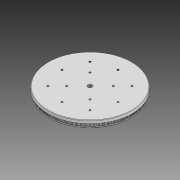
# Autodesk Inventor part: Turntable
Saved by Autodesk Inventor 2020 (Build 240168000, 168)
## iProperties
Created: 2020-10-19
Part Number: Turntable
Material: Generic
Document SubType Name: Modeling
Designer: DDeGo
Density: 1 g/cm^3
Appearance: Default
Author: DDeGo
Autodesk Inventor part; units mm, degrees
ref_plane "YZ Plane" through (0, 0, 0) normal (1, 0, 0) x (0, 1, 0)
ref_plane "XZ Plane" through (0, 0, 0) normal (0, 1, 0) x (-1, 0, 0)
ref_plane "XY Plane" through (0, 0, 0) normal (0, 0, 1) x (1, 0, 0)
sketch "Sketch1" plane through (0, 0, 0) normal (0, 0, 1) x (1, 0, 0)
  line L0 (0, 0) -> (0, 13.2) construction
  line L1 (0, 14.7) -> (90, 14.7)
  line L2 (88.5, 0) -> (73.1, 0)
  line L3 (73.1, 0) -> (73.1, 12.8)
  line L4 (0, 0) -> (73.1, 0) construction
  line L5 (0, 13.2) -> (0, 14.7)
  line L6 (90, 8.5) -> (87.5, 8.5)
  line L7 (87.5, 8.5) -> (87.5, 1.5)
  line L8 (87.5, 1.5) -> (88.5, 1.5)
  line L9 (90, 14.7) -> (90, 8.5)
  line L10 (88.5, 1.5) -> (88.5, 0)
  line L11 (73.1, 12.8) -> (69.1, 12.8)
  line L12 (69.1, 12.8) -> (69.1, 13.2)
  line L13 (69.1, 13.2) -> (0, 13.2)
  dimension "d0" = 90
  dimension "d6" = 7
  dimension "d9" = 87.5
  dimension "d11" = 1
  dimension "d12" = 1.5
  dimension "d13" = 73.1
  dimension "d14" = 12.8
  dimension "d15" = 0.4
  dimension "d16" = 4
  dimension "d17" = 1.5
  constraints: 28 end point, 9 perpendicular, 3 horizontal, 2 vertical, 1 collinear, 1 parallel
  measures "d0" distance of L1.start L1.end
  measures "d6" distance of L6.end L7.end
  measures "d9" distance between parallel lines of L7 L0
  measures "d11" distance of L7.end L8.end
  measures "d12" distance of L8.end L2.start
  measures "d13" distance between parallel lines of L0 L3
  measures "d14" distance of L2.end L3.end
  measures "d15" distance of L11.end L12.end
  measures "d16" distance of L3.end L11.end
  measures "d17" distance between parallel lines of L1 L13
revolve "Revolution1" add sketch "Sketch1" angle 360 about axis through (0, 13.2, 0) along (0, 1, 0)
sketch "Sketch3" plane through (0, 8.5, 0) normal (0, -1, 0) x (1, 0, 0)
  line L0 (0, 0) -> (87.5, 0) construction
  circle A0 centre (0, 0) radius 87.5 projected
  circle A1 centre (87.5, 0) radius 0.65
  circle A2 centre (87.478, -1.9633) radius 0.65
  circle A3 centre (87.4119, -3.9257) radius 0.65
  circle A4 centre (87.3018, -5.886) radius 0.65
  circle A5 centre (87.1478, -7.8434) radius 0.65
  circle A6 centre (86.9498, -9.7969) radius 0.65
  circle A7 centre (86.7081, -11.7454) radius 0.65
  circle A8 centre (86.4227, -13.688) radius 0.65
  circle A9 centre (86.0938, -15.6237) radius 0.65
  circle A10 centre (85.7216, -17.5516) radius 0.65
  circle A11 centre (85.3062, -19.4706) radius 0.65
  circle A12 centre (84.8478, -21.3798) radius 0.65
  circle A13 centre (84.3468, -23.2782) radius 0.65
  circle A14 centre (83.8032, -25.1649) radius 0.65
  circle A15 centre (83.2174, -27.039) radius 0.65
  circle A16 centre (82.5898, -28.8994) radius 0.65
  circle A17 centre (81.9206, -30.7453) radius 0.65
  circle A18 centre (81.2101, -32.5757) radius 0.65
  circle A19 centre (80.4587, -34.3897) radius 0.65
  circle A20 centre (79.6668, -36.1864) radius 0.65
  circle A21 centre (78.8348, -37.9648) radius 0.65
  circle A22 centre (77.9631, -39.7242) radius 0.65
  circle A23 centre (77.0521, -41.4635) radius 0.65
  circle A24 centre (76.1023, -43.182) radius 0.65
  circle A25 centre (75.1143, -44.8787) radius 0.65
  circle A26 centre (74.0884, -46.5528) radius 0.65
  circle A27 centre (73.0252, -48.2035) radius 0.65
  circle A28 centre (71.9252, -49.8299) radius 0.65
  circle A29 centre (70.789, -51.4312) radius 0.65
  circle A30 centre (69.6171, -53.0066) radius 0.65
  circle A31 centre (68.4103, -54.5554) radius 0.65
  circle A32 centre (67.1689, -56.0766) radius 0.65
  circle A33 centre (65.8938, -57.5696) radius 0.65
  circle A34 centre (64.5854, -59.0337) radius 0.65
  circle A35 centre (63.2446, -60.468) radius 0.65
  circle A36 centre (61.8718, -61.8718) radius 0.65
  circle A37 centre (60.468, -63.2446) radius 0.65
  circle A38 centre (59.0337, -64.5854) radius 0.65
  circle A39 centre (57.5696, -65.8938) radius 0.65
  circle A40 centre (56.0766, -67.1689) radius 0.65
  circle A41 centre (54.5554, -68.4103) radius 0.65
  circle A42 centre (53.0066, -69.6171) radius 0.65
  circle A43 centre (51.4312, -70.789) radius 0.65
  circle A44 centre (49.8299, -71.9252) radius 0.65
  circle A45 centre (48.2035, -73.0252) radius 0.65
  circle A46 centre (46.5528, -74.0884) radius 0.65
  circle A47 centre (44.8787, -75.1143) radius 0.65
  circle A48 centre (43.182, -76.1023) radius 0.65
  circle A49 centre (41.4635, -77.0521) radius 0.65
  circle A50 centre (39.7242, -77.9631) radius 0.65
  circle A51 centre (37.9648, -78.8348) radius 0.65
  circle A52 centre (36.1864, -79.6668) radius 0.65
  circle A53 centre (34.3897, -80.4587) radius 0.65
  circle A54 centre (32.5757, -81.2101) radius 0.65
  circle A55 centre (30.7453, -81.9206) radius 0.65
  circle A56 centre (28.8994, -82.5898) radius 0.65
  circle A57 centre (27.039, -83.2174) radius 0.65
  circle A58 centre (25.1649, -83.8032) radius 0.65
  circle A59 centre (23.2782, -84.3468) radius 0.65
  circle A60 centre (21.3798, -84.8478) radius 0.65
  circle A61 centre (19.4706, -85.3062) radius 0.65
  circle A62 centre (17.5516, -85.7216) radius 0.65
  circle A63 centre (15.6237, -86.0938) radius 0.65
  circle A64 centre (13.688, -86.4227) radius 0.65
  circle A65 centre (11.7454, -86.7081) radius 0.65
  circle A66 centre (9.7969, -86.9498) radius 0.65
  circle A67 centre (7.8434, -87.1478) radius 0.65
  circle A68 centre (5.886, -87.3018) radius 0.65
  circle A69 centre (3.9257, -87.4119) radius 0.65
  circle A70 centre (1.9633, -87.478) radius 0.65
  circle A71 centre (0, -87.5) radius 0.65
  circle A72 centre (-1.9633, -87.478) radius 0.65
  circle A73 centre (-3.9257, -87.4119) radius 0.65
  circle A74 centre (-5.886, -87.3018) radius 0.65
  circle A75 centre (-7.8434, -87.1478) radius 0.65
  circle A76 centre (-9.7969, -86.9498) radius 0.65
  circle A77 centre (-11.7454, -86.7081) radius 0.65
  circle A78 centre (-13.688, -86.4227) radius 0.65
  circle A79 centre (-15.6237, -86.0938) radius 0.65
  circle A80 centre (-17.5516, -85.7216) radius 0.65
  circle A81 centre (-19.4706, -85.3062) radius 0.65
  circle A82 centre (-21.3798, -84.8478) radius 0.65
  circle A83 centre (-23.2782, -84.3468) radius 0.65
  circle A84 centre (-25.1649, -83.8032) radius 0.65
  circle A85 centre (-27.039, -83.2174) radius 0.65
  circle A86 centre (-28.8994, -82.5898) radius 0.65
  circle A87 centre (-30.7453, -81.9206) radius 0.65
  circle A88 centre (-32.5757, -81.2101) radius 0.65
  circle A89 centre (-34.3897, -80.4587) radius 0.65
  circle A90 centre (-36.1864, -79.6668) radius 0.65
  circle A91 centre (-37.9648, -78.8348) radius 0.65
  circle A92 centre (-39.7242, -77.9631) radius 0.65
  circle A93 centre (-41.4635, -77.0521) radius 0.65
  circle A94 centre (-43.182, -76.1023) radius 0.65
  circle A95 centre (-44.8787, -75.1143) radius 0.65
  circle A96 centre (-46.5528, -74.0884) radius 0.65
  circle A97 centre (-48.2035, -73.0252) radius 0.65
  circle A98 centre (-49.8299, -71.9252) radius 0.65
  circle A99 centre (-51.4312, -70.789) radius 0.65
  circle A100 centre (-53.0066, -69.6171) radius 0.65
  circle A101 centre (-54.5554, -68.4103) radius 0.65
  circle A102 centre (-56.0766, -67.1689) radius 0.65
  circle A103 centre (-57.5696, -65.8938) radius 0.65
  circle A104 centre (-59.0337, -64.5854) radius 0.65
  circle A105 centre (-60.468, -63.2446) radius 0.65
  circle A106 centre (-61.8718, -61.8718) radius 0.65
  circle A107 centre (-63.2446, -60.468) radius 0.65
  circle A108 centre (-64.5854, -59.0337) radius 0.65
  circle A109 centre (-65.8938, -57.5696) radius 0.65
  circle A110 centre (-67.1689, -56.0766) radius 0.65
  circle A111 centre (-68.4103, -54.5554) radius 0.65
  circle A112 centre (-69.6171, -53.0066) radius 0.65
  circle A113 centre (-70.789, -51.4312) radius 0.65
  circle A114 centre (-71.9252, -49.8299) radius 0.65
  circle A115 centre (-73.0252, -48.2035) radius 0.65
  circle A116 centre (-74.0884, -46.5528) radius 0.65
  circle A117 centre (-75.1143, -44.8787) radius 0.65
  circle A118 centre (-76.1023, -43.182) radius 0.65
  circle A119 centre (-77.0521, -41.4635) radius 0.65
  circle A120 centre (-77.9631, -39.7242) radius 0.65
  circle A121 centre (-78.8348, -37.9648) radius 0.65
  circle A122 centre (-79.6668, -36.1864) radius 0.65
  circle A123 centre (-80.4587, -34.3897) radius 0.65
  circle A124 centre (-81.2101, -32.5757) radius 0.65
  circle A125 centre (-81.9206, -30.7453) radius 0.65
  circle A126 centre (-82.5898, -28.8994) radius 0.65
  circle A127 centre (-83.2174, -27.039) radius 0.65
  circle A128 centre (-83.8032, -25.1649) radius 0.65
  circle A129 centre (-84.3468, -23.2782) radius 0.65
  circle A130 centre (-84.8478, -21.3798) radius 0.65
  circle A131 centre (-85.3062, -19.4706) radius 0.65
  circle A132 centre (-85.7216, -17.5516) radius 0.65
  circle A133 centre (-86.0938, -15.6237) radius 0.65
  circle A134 centre (-86.4227, -13.688) radius 0.65
  circle A135 centre (-86.7081, -11.7454) radius 0.65
  circle A136 centre (-86.9498, -9.7969) radius 0.65
  circle A137 centre (-87.1478, -7.8434) radius 0.65
  circle A138 centre (-87.3018, -5.886) radius 0.65
  circle A139 centre (-87.4119, -3.9257) radius 0.65
  circle A140 centre (-87.478, -1.9633) radius 0.65
  circle A141 centre (-87.5, 0) radius 0.65
  circle A142 centre (-87.478, 1.9633) radius 0.65
  circle A143 centre (-87.4119, 3.9257) radius 0.65
  circle A144 centre (-87.3018, 5.886) radius 0.65
  circle A145 centre (-87.1478, 7.8434) radius 0.65
  circle A146 centre (-86.9498, 9.7969) radius 0.65
  circle A147 centre (-86.7081, 11.7454) radius 0.65
  circle A148 centre (-86.4227, 13.688) radius 0.65
  circle A149 centre (-86.0938, 15.6237) radius 0.65
  circle A150 centre (-85.7216, 17.5516) radius 0.65
  circle A151 centre (-85.3062, 19.4706) radius 0.65
  circle A152 centre (-84.8478, 21.3798) radius 0.65
  circle A153 centre (-84.3468, 23.2782) radius 0.65
  circle A154 centre (-83.8032, 25.1649) radius 0.65
  circle A155 centre (-83.2174, 27.039) radius 0.65
  circle A156 centre (-82.5898, 28.8994) radius 0.65
  circle A157 centre (-81.9206, 30.7453) radius 0.65
  circle A158 centre (-81.2101, 32.5757) radius 0.65
  circle A159 centre (-80.4587, 34.3897) radius 0.65
  circle A160 centre (-79.6668, 36.1864) radius 0.65
  circle A161 centre (-78.8348, 37.9648) radius 0.65
  circle A162 centre (-77.9631, 39.7242) radius 0.65
  circle A163 centre (-77.0521, 41.4635) radius 0.65
  circle A164 centre (-76.1023, 43.182) radius 0.65
  circle A165 centre (-75.1143, 44.8787) radius 0.65
  circle A166 centre (-74.0884, 46.5528) radius 0.65
  circle A167 centre (-73.0252, 48.2035) radius 0.65
  circle A168 centre (-71.9252, 49.8299) radius 0.65
  circle A169 centre (-70.789, 51.4312) radius 0.65
  circle A170 centre (-69.6171, 53.0066) radius 0.65
  circle A171 centre (-68.4103, 54.5554) radius 0.65
  circle A172 centre (-67.1689, 56.0766) radius 0.65
  circle A173 centre (-65.8938, 57.5696) radius 0.65
  circle A174 centre (-64.5854, 59.0337) radius 0.65
  circle A175 centre (-63.2446, 60.468) radius 0.65
  circle A176 centre (-61.8718, 61.8718) radius 0.65
  circle A177 centre (-60.468, 63.2446) radius 0.65
  circle A178 centre (-59.0337, 64.5854) radius 0.65
  circle A179 centre (-57.5696, 65.8938) radius 0.65
  circle A180 centre (-56.0766, 67.1689) radius 0.65
  circle A181 centre (-54.5554, 68.4103) radius 0.65
  circle A182 centre (-53.0066, 69.6171) radius 0.65
  circle A183 centre (-51.4312, 70.789) radius 0.65
  circle A184 centre (-49.8299, 71.9252) radius 0.65
  circle A185 centre (-48.2035, 73.0252) radius 0.65
  circle A186 centre (-46.5528, 74.0884) radius 0.65
  circle A187 centre (-44.8787, 75.1143) radius 0.65
  circle A188 centre (-43.182, 76.1023) radius 0.65
  circle A189 centre (-41.4635, 77.0521) radius 0.65
  circle A190 centre (-39.7242, 77.9631) radius 0.65
  circle A191 centre (-37.9648, 78.8348) radius 0.65
  circle A192 centre (-36.1864, 79.6668) radius 0.65
  circle A193 centre (-34.3897, 80.4587) radius 0.65
  circle A194 centre (-32.5757, 81.2101) radius 0.65
  circle A195 centre (-30.7453, 81.9206) radius 0.65
  circle A196 centre (-28.8994, 82.5898) radius 0.65
  circle A197 centre (-27.039, 83.2174) radius 0.65
  circle A198 centre (-25.1649, 83.8032) radius 0.65
  circle A199 centre (-23.2782, 84.3468) radius 0.65
  circle A200 centre (-21.3798, 84.8478) radius 0.65
  circle A201 centre (-19.4706, 85.3062) radius 0.65
  circle A202 centre (-17.5516, 85.7216) radius 0.65
  circle A203 centre (-15.6237, 86.0938) radius 0.65
  circle A204 centre (-13.688, 86.4227) radius 0.65
  circle A205 centre (-11.7454, 86.7081) radius 0.65
  circle A206 centre (-9.7969, 86.9498) radius 0.65
  circle A207 centre (-7.8434, 87.1478) radius 0.65
  circle A208 centre (-5.886, 87.3018) radius 0.65
  circle A209 centre (-3.9257, 87.4119) radius 0.65
  circle A210 centre (-1.9633, 87.478) radius 0.65
  circle A211 centre (0, 87.5) radius 0.65
  circle A212 centre (1.9633, 87.478) radius 0.65
  circle A213 centre (3.9257, 87.4119) radius 0.65
  circle A214 centre (5.886, 87.3018) radius 0.65
  circle A215 centre (7.8434, 87.1478) radius 0.65
  circle A216 centre (9.7969, 86.9498) radius 0.65
  circle A217 centre (11.7454, 86.7081) radius 0.65
  circle A218 centre (13.688, 86.4227) radius 0.65
  circle A219 centre (15.6237, 86.0938) radius 0.65
  circle A220 centre (17.5516, 85.7216) radius 0.65
  circle A221 centre (19.4706, 85.3062) radius 0.65
  circle A222 centre (21.3798, 84.8478) radius 0.65
  circle A223 centre (23.2782, 84.3468) radius 0.65
  circle A224 centre (25.1649, 83.8032) radius 0.65
  circle A225 centre (27.039, 83.2174) radius 0.65
  circle A226 centre (28.8994, 82.5898) radius 0.65
  circle A227 centre (30.7453, 81.9206) radius 0.65
  circle A228 centre (32.5757, 81.2101) radius 0.65
  circle A229 centre (34.3897, 80.4587) radius 0.65
  circle A230 centre (36.1864, 79.6668) radius 0.65
  circle A231 centre (37.9648, 78.8348) radius 0.65
  circle A232 centre (39.7242, 77.9631) radius 0.65
  circle A233 centre (41.4635, 77.0521) radius 0.65
  circle A234 centre (43.182, 76.1023) radius 0.65
  circle A235 centre (44.8787, 75.1143) radius 0.65
  circle A236 centre (46.5528, 74.0884) radius 0.65
  circle A237 centre (48.2035, 73.0252) radius 0.65
  circle A238 centre (49.8299, 71.9252) radius 0.65
  circle A239 centre (51.4312, 70.789) radius 0.65
  circle A240 centre (53.0066, 69.6171) radius 0.65
  circle A241 centre (54.5554, 68.4103) radius 0.65
  circle A242 centre (56.0766, 67.1689) radius 0.65
  circle A243 centre (57.5696, 65.8938) radius 0.65
  circle A244 centre (59.0337, 64.5854) radius 0.65
  circle A245 centre (60.468, 63.2446) radius 0.65
  circle A246 centre (61.8718, 61.8718) radius 0.65
  circle A247 centre (63.2446, 60.468) radius 0.65
  circle A248 centre (64.5854, 59.0337) radius 0.65
  circle A249 centre (65.8938, 57.5696) radius 0.65
  circle A250 centre (67.1689, 56.0766) radius 0.65
  circle A251 centre (68.4103, 54.5554) radius 0.65
  circle A252 centre (69.6171, 53.0066) radius 0.65
  circle A253 centre (70.789, 51.4312) radius 0.65
  circle A254 centre (71.9252, 49.8299) radius 0.65
  circle A255 centre (73.0252, 48.2035) radius 0.65
  circle A256 centre (74.0884, 46.5528) radius 0.65
  circle A257 centre (75.1143, 44.8787) radius 0.65
  circle A258 centre (76.1023, 43.182) radius 0.65
  circle A259 centre (77.0521, 41.4635) radius 0.65
  circle A260 centre (77.9631, 39.7242) radius 0.65
  circle A261 centre (78.8348, 37.9648) radius 0.65
  circle A262 centre (79.6668, 36.1864) radius 0.65
  circle A263 centre (80.4587, 34.3897) radius 0.65
  circle A264 centre (81.2101, 32.5757) radius 0.65
  circle A265 centre (81.9206, 30.7453) radius 0.65
  circle A266 centre (82.5898, 28.8994) radius 0.65
  circle A267 centre (83.2174, 27.039) radius 0.65
  circle A268 centre (83.8032, 25.1649) radius 0.65
  circle A269 centre (84.3468, 23.2782) radius 0.65
  circle A270 centre (84.8478, 21.3798) radius 0.65
  circle A271 centre (85.3062, 19.4706) radius 0.65
  circle A272 centre (85.7216, 17.5516) radius 0.65
  circle A273 centre (86.0938, 15.6237) radius 0.65
  circle A274 centre (86.4227, 13.688) radius 0.65
  circle A275 centre (86.7081, 11.7454) radius 0.65
  circle A276 centre (86.9498, 9.7969) radius 0.65
  circle A277 centre (87.1478, 7.8434) radius 0.65
  circle A278 centre (87.3018, 5.886) radius 0.65
  circle A279 centre (87.4119, 3.9257) radius 0.65
  circle A280 centre (87.478, 1.9633) radius 0.65
  dimension "d19" = 1.3
  dimension "d22" = 360
  dimension "d24" = 1.9633
  constraints: 280 centre point, 2 end point, 1 coincident, 1 horizontal, 1 horizontal alignment, 562 other
  measures "d19" diameter of A1
  measures "d24" vertical distance of A2.centre L0.end
extrude "Extrusion1" cut sketch "Sketch3" along normal up to surface (7 mm away) contours A0 A1 | A0 A1 | A280 A0 | A0 A280 | A2 A0 | A0 A2 | A279 A0 | A0 A279 | A3 A0 | A0 A3 | A278 A0 | A0 A278 | A4 A0 | A0 A4 | A277 A0 | A0 A277 | A5 A0 | A0 A5 | A276 A0 | A0 A276 | A6 A0 | A0 A6 | A275 A0 | A0 A275 | A7 A0 | A0 A7 | A274 A0 | A0 A274 | A8 A0 | A0 A8 | A273 A0 | A0 A273 | A9 A0 | A0 A9 | A272 A0 | A0 A272 | A10 A0 | A0 A10 | A271 A0 | A0 A271 | A11 A0 | A0 A11 | A270 A0 | A0 A270 | A12 A0 | A0 A12 | A269 A0 | A0 A269 | A13 A0 | A0 A13 | A268 A0 | A0 A268 | A14 A0 | A0 A14 | A267 A0 | A0 A267 | A15 A0 | A0 A15 | A266 A0 | A0 A266 | A16 A0 | A0 A16 | A265 A0 | A0 A265 | A17 A0 | A0 A17 | A264 A0 | A0 A264 | A18 A0 | A0 A18 | A263 A0 | A0 A263 | A19 A0 | A0 A19 | A262 A0 | A0 A262 | A20 A0 | A0 A20 | A261 A0 | A0 A261 | A21 A0 | A0 A21 | A260 A0 | A0 A260 | A22 A0 | A0 A22 | A259 A0 | A0 A259 | A23 A0 | A0 A23 | A258 A0 | A0 A258 | A24 A0 | A0 A24 | A257 A0 | A0 A257 | A25 A0 | A0 A25 | A256 A0 | A0 A256 | A26 A0 | A0 A26 | A255 A0 | A0 A255 | A27 A0 | A0 A27 | A254 A0 | A0 A254 | A28 A0 | A0 A28 | A253 A0 | A0 A253 | A29 A0 | A0 A29 | A252 A0 | A0 A252 | A30 A0 | A0 A30 | A251 A0 | A0 A251 | A31 A0 | A0 A31 | A250 A0 | A0 A250 | A32 A0 | A0 A32 | A249 A0 | A0 A249 | A33 A0 | A0 A33 | A248 A0 | A0 A248 | A34 A0 | A0 A34 | A247 A0 | A0 A247 | A35 A0 | A0 A35 | A246 A0 | A0 A246 | A36 A0 | A0 A36 | A245 A0 | A0 A245 | A37 A0 | A0 A37 | A244 A0 | A0 A244 | A38 A0 | A0 A38 | A243 A0 | A0 A243 | A39 A0 | A0 A39 | A242 A0 | A0 A242 | A40 A0 | A0 A40 | A241 A0 | A0 A241 | A41 A0 | A0 A41 | A240 A0 | A0 A240 | A42 A0 | A0 A42 | A239 A0 | A0 A239 | A43 A0 | A0 A43 | A238 A0 | A0 A238 | A44 A0 | A0 A44 | A237 A0 | A0 A237 | A45 A0 | A0 A45 | A236 A0 | A0 A236 | A46 A0 | A0 A46 | A235 A0 | A0 A235 | A47 A0 | A0 A47 | A234 A0 | A0 A234 | A48 A0 | A0 A48 | A233 A0 | A0 A233 | A49 A0 | A0 A49 | A232 A0 | A0 A232 | A50 A0 | A0 A50 | A231 A0 | A0 A231 | A51 A0 | A0 A51 | A230 A0 | A0 A230 | A52 A0 | A0 A52 | A229 A0 | A0 A229 | A53 A0 | A0 A53 | A228 A0 | A0 A228 | A54 A0 | A0 A54 | A227 A0 | A0 A227 | A55 A0 | A0 A55 | A226 A0 | A0 A226 | A56 A0 | A0 A56 | A225 A0 | A0 A225 | A57 A0 | A0 A57 | A224 A0 | A0 A224 | A58 A0 | A0 A58 | A223 A0 | A0 A223 | A59 A0 | A0 A59 | A222 A0 | A0 A222 | A60 A0 | A0 A60 | A221 A0 | A0 A221 | A61 A0 | A0 A61 | A220 A0 | A0 A220 | A62 A0 | A0 A62 | A219 A0 | A0 A219 | A63 A0 | A0 A63 | A218 A0 | A0 A218 | A64 A0 | A0 A64 | A217 A0 | A0 A217 | A65 A0 | A0 A65 | A216 A0 | A0 A216 | A66 A0 | A0 A66 | A215 A0 | A0 A215 | A67 A0 | A0 A67 | A214 A0 | A0 A214 | A68 A0 | A0 A68 | A213 A0 | A0 A213 | A69 A0 | A0 A69 | A212 A0 | A0 A212 | A70 A0 | A0 A70 | A211 A0 | A0 A211 | A71 A0 | A0 A71 | A210 A0 | A0 A210 | A72 A0 | A0 A72 | A209 A0 | A0 A209 | A73 A0 | A0 A73 | A208 A0 | A0 A208 | A74 A0 | A0 A74 | A207 A0 | A0 A207 | A75 A0 | A0 A75 | A206 A0 | A0 A206 | A76 A0 | A0 A76 | A205 A0 | A0 A205 | A77 A0 | A0 A77 | A204 A0 | A0 A204 | A78 A0 | A0 A78 | A203 A0 | A0 A203 | A79 A0 | A0 A79 | A202 A0 | A0 A202 | A80 A0 | A0 A80 | A201 A0 | A0 A201 | A81 A0 | A0 A81 | A200 A0 | A0 A200 | A82 A0 | A0 A82 | A199 A0 | A0 A199 | A83 A0 | A0 A83 | A198 A0 | A0 A198 | A84 A0 | A0 A84 | A197 A0 | A0 A197 | A85 A0 | A0 A85 | A196 A0 | A0 A196 | A86 A0 | A0 A86 | A195 A0 | A0 A195 | A87 A0 | A0 A87 | A194 A0 | A0 A194 | A88 A0 | A0 A88 | A193 A0 | A0 A193 | A89 A0 | A0 A89 | A192 A0 | A0 A192 | A90 A0 | A0 A90 | A191 A0 | A0 A191 | A91 A0 | A0 A91 | A190 A0 | A0 A190 | A92 A0 | A0 A92 | A189 A0 | A0 A189 | A93 A0 | A0 A93 | A188 A0 | A0 A188 | A94 A0 | A0 A94 | A187 A0 | A0 A187 | A95 A0 | A0 A95 | A186 A0 | A0 A186 | A96 A0 | A0 A96 | A185 A0 | A0 A185 | A97 A0 | A0 A97 | A184 A0 | A0 A184 | A98 A0 | A0 A98 | A183 A0 | A0 A183 | A99 A0 | A0 A99 | A182 A0 | A0 A182 | A100 A0 | A0 A100 | A181 A0 | A0 A181 | A101 A0 | A0 A101 | A180 A0 | A0 A180 | A102 A0 | A0 A102 | A179 A0 | A0 A179 | A103 A0 | A0 A103 | A178 A0 | A0 A178 | A104 A0 | A0 A104 | A177 A0 | A0 A177 | A105 A0 | A0 A105 | A176 A0 | A0 A176 | A106 A0 | A0 A106 | A175 A0 | A0 A175 | A107 A0 | A0 A107 | A174 A0 | A0 A174 | A108 A0 | A0 A108 | A173 A0 | A0 A173 | A109 A0 | A0 A109 | A172 A0 | A0 A172 | A110 A0 | A0 A110 | A171 A0 | A0 A171 | A111 A0 | A0 A111 | A170 A0 | A0 A170 | A112 A0 | A0 A112 | A169 A0 | A0 A169 | A113 A0 | A0 A113 | A168 A0 | A0 A168 | A114 A0 | A0 A114 | A167 A0 | A0 A167 | A115 A0 | A0 A115 | A166 A0 | A0 A166 | A116 A0 | A0 A116 | A165 A0 | A0 A165 | A117 A0 | A0 A117 | A164 A0 | A0 A164 | A118 A0 | A0 A118 | A163 A0 | A0 A163 | A119 A0 | A0 A119 | A162 A0 | A0 A162 | A120 A0 | A0 A120 | A161 A0 | A0 A161 | A121 A0 | A0 A121 | A160 A0 | A0 A160 | A122 A0 | A0 A122 | A159 A0 | A0 A159 | A123 A0 | A0 A123 | A158 A0 | A0 A158 | A124 A0 | A0 A124 | A157 A0 | A0 A157 | A125 A0 | A0 A125 | A156 A0 | A0 A156 | A126 A0 | A0 A126 | A155 A0 | A0 A155 | A127 A0 | A0 A127 | A154 A0 | A0 A154 | A128 A0 | A0 A128 | A153 A0 | A0 A153 | A129 A0 | A0 A129 | A152 A0 | A0 A152 | A130 A0 | A0 A130 | A151 A0 | A0 A151 | A131 A0 | A0 A131 | A150 A0 | A0 A150 | A132 A0 | A0 A132 | A149 A0 | A0 A149 | A133 A0 | A0 A133 | A148 A0 | A0 A148 | A134 A0 | A0 A134 | A147 A0 | A0 A147 | A135 A0 | A0 A135 | A146 A0 | A0 A146 | A136 A0 | A0 A136 | A145 A0 | A0 A145 | A137 A0 | A0 A137 | A144 A0 | A0 A144 | A138 A0 | A0 A138 | A143 A0 | A0 A143 | A139 A0 | A0 A139 | A142 A0 | A0 A142 | A140 A0 | A0 A140 | A141 A0 | A0 A141
chamfer "Chamfer1" distance 2 angle 45 1 edges at (-73.1, 0, 0)
chamfer "Chamfer2" distance 1 angle 45 1 edges at (-90, 14.7, 0)
chamfer "Chamfer3" distance 1 angle 45 1 edges at (-88.5, 1.5, 0)
sketch "Sketch5" plane through (0, 13.2, 0) normal (0, -1, 0) x (1, 0, 0)
  line L0 (-25, 25) -> (25, 25) construction
  line L1 (25, 25) -> (25, -25) construction
  line L2 (25, -25) -> (-25, -25) construction
  line L3 (-25, -25) -> (-25, 25) construction
  line L4 (-25, 25) -> (25, -25) construction
  line L5 (25, 25) -> (-25, -25) construction
  line L6 (-60, 60) -> (60, 60) construction
  line L7 (60, 60) -> (60, -60) construction
  line L8 (60, -60) -> (-60, -60) construction
  line L9 (-60, -60) -> (-60, 60) construction
  line L10 (-60, 60) -> (60, -60) construction
  line L11 (60, 60) -> (-60, -60) construction
  line L12 (45, -45) -> (-45, -45) construction
  line L13 (-45, -45) -> (-45, 45) construction
  line L14 (-45, 45) -> (45, 45) construction
  line L15 (45, 45) -> (45, -45) construction
  line L16 (45, -45) -> (-45, 45) construction
  line L17 (-45, -45) -> (45, 45) construction
  point P0 (0, 0)
  point P1 (60, 0)
  point P2 (0, 60)
  point P3 (0, -60)
  point P4 (-60, 0)
  dimension "d51" = 120
  dimension "d52" = 50
  dimension "d53" = 90
  constraints: 36 end point, 10 midpoint, 7 coincident, 6 parallel, 5 perpendicular, 3 horizontal, 1 point on line
  measures "d51" distance of L6.end L7.end
  measures "d52" distance of L0.end L1.end
  measures "d53" distance of L13.end L14.end
hole "Hole2" at (60, 13.2, 0) at (25, 13.2, 25) at (25, 13.2, -25) at (0, 13.2, 60) at (0, 13.2, -60) at (-25, 13.2, 25) at (-25, 13.2, -25) at (-60, 13.2, 0) at (-45, 13.2, 45) at (45, 13.2, 45) at (-45, 13.2, -45) at (45, 13.2, -45) direction (0, 1, 0) diameter 3 end through all countersink diameter 6.5 countersink angle 82
sketch "Sketch6" plane through (0, 13.2, 0) normal (0, -1, 0) x (1, 0, 0)
  circle A0 centre (0, 0) radius 6
  dimension "d54" = 12
  constraints: 1 centre point, 1 coincident
  measures "d54" diameter of A0
extrude "Extrusion2" add sketch "Sketch6" along normal blind 2.5
sketch "Sketch7" plane through (0, 10.7, 0) normal (0, -1, 0) x (1, 0, 0)
  circle A0 centre (0, 0) radius 2.75
  point P0 (0, 0)
  dimension "d57" = 5.5
  constraints: 1 centre point, 1 coincident
  measures "d57" diameter of A0
extrude "Extrusion3" cut sketch "Sketch7" against normal through all
sketch "Sketch8" plane through (0, 14.7, 0) normal (0, 1, 0) x (1, 0, 0)
  line L0 (4.792, 0) -> (2.396, -4.15)
  line L1 (2.396, -4.15) -> (-2.396, -4.15)
  line L2 (-2.396, -4.15) -> (-4.792, 0)
  line L3 (-4.792, 0) -> (-2.396, 4.15)
  line L4 (-2.396, 4.15) -> (2.396, 4.15)
  line L5 (2.396, 4.15) -> (4.792, 0)
  point P0 (0, 0)
  point P1 (0, 0)
  dimension "d60" = 8.3
  constraints: 12 end point, 1 coincident, 1 horizontal, 13 other
  measures "d60" distance between parallel lines of L1 L4
extrude "Extrusion4" cut sketch "Sketch8" against normal blind 2.8
chamfer "Chamfer4" distance 2.5 angle 45 1 edges at (-6, 13.2, 0)
body "Solid1"
